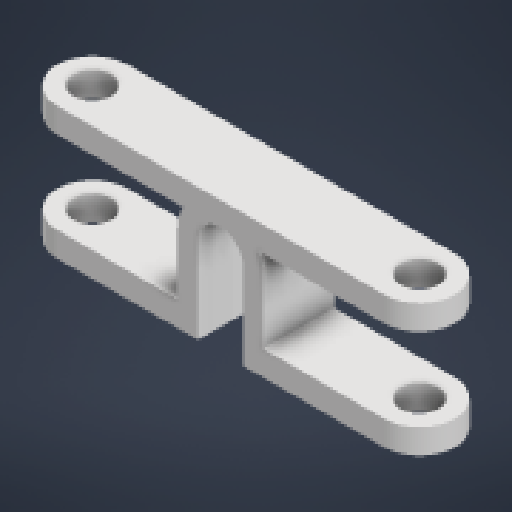
# Autodesk Inventor part: Чертёж
Saved by Autodesk Inventor 2026.2 (Build 302298000, 298)
## iProperties
Created: 2026-02-19
Part Number: Чертёж
Material: Типовые
Document SubType Name: Modeling
Designer: Leonid
Density: 1 g/cm^3
Appearance: По умолчанию
Author: Leonid
Autodesk Inventor part; units mm, degrees
ref_plane "YZ Plane" through (0, 0, 0) normal (1, 0, 0) x (0, 1, 0)
ref_plane "XZ Plane" through (0, 0, 0) normal (0, 1, 0) x (-1, 0, 0)
ref_plane "XY Plane" through (0, 0, 0) normal (0, 0, 1) x (1, 0, 0)
sketch "Эскиз1" plane through (0, 0, 0) normal (0, 1, 0) x (-1, 0, 0)
  line L0 (11.5, 0) -> (-11.5, 0) construction
  line L1 (11.5, 2.5) -> (-11.5, 2.5)
  line L2 (-11.5, -2.5) -> (11.5, -2.5)
  arc A0 (11.5, -2.5) -> (11.5, 2.5) centre (11.5, 0) ccw
  arc A1 (-11.5, 2.5) -> (-11.5, -2.5) centre (-11.5, 0) ccw
  circle A2 centre (11.5, 0) radius 1.325
  circle A3 centre (-11.5, 0) radius 1.325
  line L3 (16.5, 7.5) -> (-6.5, 7.5)
  line L4 (-6.5, 2.5) -> (16.5, 2.5)
  arc A4 (16.5, 2.5) -> (16.5, 7.5) centre (16.5, 5) ccw
  arc A5 (-6.5, 7.5) -> (-6.5, 2.5) centre (-6.5, 5) ccw
  line L5 (11.5, 0) -> (16.5, 5) construction
  point P0 (0, 0)
  point P1 (0, 0)
  point P2 (-14, 0)
  point P3 (14, 0)
  point P4 (-9, 5)
  point P5 (19, 5)
  dimension "d0" = 2.65
  dimension "d1" = 2.65
  dimension "d2" = 2.5
  dimension "d6" = 2.5
  dimension "d12" = 45
  dimension "d16" = 23
  dimension "d28" = 5
  dimension "d29" = 7.0711
  constraints: 14 end point, 12 point on circle, 8 tangent, 6 centre point, 4 coincident, 3 parallel, 1 collinear, 1 horizontal, 1 midpoint
  measures "d0" diameter of A2
  measures "d1" diameter of A3
  measures "d2" radius of A0
  measures "d6" radius of A4
  measures "d12" angle of L0 L5
  measures "d16" distance of L0.end L0.start
  measures "d28" horizontal distance of A4.centre L0.start
  measures "d29" distance of L5.start L5.end
extrude "Выдавливание1" add sketch "Эскиз1" along normal blind 1.75 contours A0 L2 A1 L1
pattern_linear "Прямоуг.массив1" count 2 spacing 7.55 along (0, 1, 0) of "Выдавливание1"
sketch "Эскиз2" plane through (0, 0, 0) normal (0, 0, 1) x (1, 0, 0)
  arc A0 (1.575, 6.1) -> (-1.575, 6.1) centre (0, 6.1) ccw
  line L0 (-11.5, 9.3) -> (11.5, 9.3) projected
  line L1 (-11.5, 0) -> (11.5, 0) projected
  line L2 (-1.575, 6.1) -> (-1.575, 0)
  line L3 (1.575, 6.1) -> (1.575, 0)
  line L4 (11.5, 7.55) -> (-11.5, 7.55) projected
  line L5 (-3.25, 7.55) -> (-3.25, 0)
  line L6 (3.25, 7.55) -> (3.25, 0)
  line L7 (0, -1.86) -> (0, 11.16) construction
  point P0 (0.6149, 7.55)
  point P1 (-0.6149, 7.55)
  dimension "d21" = 3.15
  dimension "d33" = 3.2
  dimension "d34" = 3.25
  dimension "d35" = 3.25
  constraints: 8 end point, 6 point on line, 4 perpendicular, 2 point on circle, 2 tangent, 1 centre point
  measures "d21" diameter of A0
  measures "d33" distance from line of L0 A0.centre
  measures "d34" distance from line of L6 A0.centre
  measures "d35" distance from line of L5 A0.centre
extrude "Выдавливание2" cut sketch "Эскиз2" along normal mid plane 5 contours L3 L1 L2 A0 L4 | L4 A0
extrude "Выдавливание3" add sketch "Эскиз2" along normal mid plane 5 contours A0 L4 L6 L1 L3 | A0 L2 L1 L5 L4
